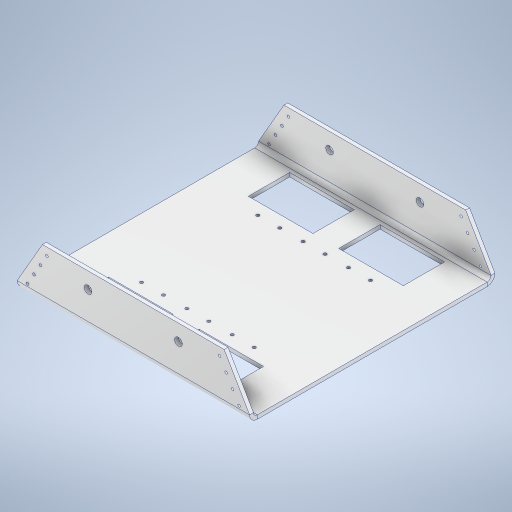
# Autodesk Inventor part: floor
Saved by Autodesk Inventor 2023 (Build 270158000, 158)
## iProperties
Created: 2022-05-09
Part Number: floor
Material: Aluminum 6061
Document SubType Name: Sheet Metal
Designer: Dan
Density: 2.7 g/cm^3
Sheet Metal Rule: Default_mm
Appearance: Aluminum - Flat
Mass: 314.843 g
Surface Area: 829.813 cm^2
Volume: 116.609 cm^3
Flat Pattern Width: 18 cm
Flat Pattern Length: 25.9572 cm
Flat Pattern Area: 467.229 cm^2
Sheet Metal Width: 180.000 mm
Sheet Metal Length: 259.572 mm
Sheet Metal Area: 46722.902 mm^2
Author: Dan
Autodesk Inventor part; units mm, degrees
ref_plane "YZ Plane" through (0, 0, 0) normal (1, 0, 0) x (0, 1, 0)
ref_plane "XZ Plane" through (0, 0, 0) normal (0, 1, 0) x (-1, 0, 0)
ref_plane "XY Plane" through (0, 0, 0) normal (0, 0, 1) x (1, 0, 0)
sketch "Sketch1" plane through (0, 0, 0) normal (0, 1, 0) x (-1, 0, 0)
  line L0 (0, 0) -> (90, 0)
  line L1 (90, 0) -> (90, -92)
  line L2 (90, -92) -> (0, -92)
  line L3 (0, -92) -> (0, 0)
  dimension "d0" = 92
  dimension "d1" = 90
  measures "d0" distance of L0.end L1.end
  measures "d1" distance of L1.end L2.end
extrude "Plate1" add sketch "Sketch1" along normal blind 3
sketch "Sketch2" plane through (0, 3, 0) normal (0, 0, 1) x (1, 0, 0)
  line L0 (-90, 0) -> (0, 0)
  line L1 (0, 0) -> (0, 37)
  line L2 (0, 37) -> (-90, 37)
  line L3 (-90, 37) -> (-90, 0)
  constraints: 6 end point, 1 horizontal, 1 perpendicular, 1 vertical
edge flange "Flange1" height 40 angle 90 thickness 3 bend radius 3 thickness toward (0, 0, 1) relief straight relief width 3 relief depth 1.5 edges at (-45, 3, 0) wall of the first edge with corners at (-90, 3, 0) (0, 3, 0) (0, 40, 0) (-90, 40, 0)
bend "Bend1"
corner "Corner1"
sketch "Sketch5" plane through (0, 3, 0) normal (0, 1, 0) x (1, 0, 0)
  line L0 (-80, 37.8978) -> (-30, 37.8978)
  line L1 (-30, 37.8978) -> (-30, 5.8978)
  line L2 (-30, 5.8978) -> (-80, 5.8978)
  line L3 (-80, 5.8978) -> (-80, 37.8978)
  line L4 (8.7792, 47.5) -> (-90, 47.5) construction
  line L5 (-90, 3) -> (-90, 92) projected
  line L6 (0, 92) -> (0, 3) projected
  line L7 (-55, 5.8978) -> (-55, 37.8978) construction
  point P0 (0, 0)
  dimension "d45" = 32
  dimension "d46" = 50
  dimension "d81" = 35
  constraints: 12 end point, 3 midpoint, 2 horizontal, 2 parallel, 1 perpendicular
  measures "d45" distance of L2.end L0.start
  measures "d46" distance of L1.end L2.end
  measures "d81" distance between parallel lines of L7 L5
extrude "Cut2" cut sketch "Sketch5" against normal blind 3
sketch "Sketch7" plane through (0, 3, 0) normal (0, 1, 0) x (1, 0, 0)
  line L0 (-90, 3) -> (-90, 92) projected
  line L1 (-80, 5.8978) -> (-80, 37.8978) projected
  line L2 (-80, 21.8978) -> (-101.6917, 21.8978) construction
  line L3 (-63.3842, 47) -> (-46.3842, 47) construction
  line L4 (-30, 37.8978) -> (-80, 37.8978) projected
  line L5 (-90, 92) -> (0, 92) projected
  point P0 (0, 0)
  point P1 (-81.5, 47)
  dimension "d88" = 17
  dimension "d90" = 45
  constraints: 4 end point, 2 horizontal, 1 horizontal alignment, 1 midpoint
  measures "d88" distance of L3.start L3.end
  measures "d90" distance from line of L5 point (-81.5, 47)
hole "Hole2" at (-46.3842, 3, -47) at (-63.3842, 3, -47) at (-81.5, 3, -47) direction (0, -1, 0) diameter 2.459 end through all thread size "M3x0.5" class "6H" standard "ISO Metric profile"
sketch "Sketch4" plane through (-15, 0, 3) normal (0, 0, 1) x (1, 0, 0)
  circle A0 centre (6.906, 8.0192) radius 1
  line L0 (17.454, -10.2505) -> (-9.0222, 35.6077) construction
  circle A1 centre (1.906, 16.6795) radius 1
  circle A2 centre (-3.094, 25.3397) radius 1
  circle A3 centre (-8.094, 34) radius 1
  line L1 (15, 0) -> (-75, 0) projected
  line L2 (15, 6) -> (15, 3) projected
  line L3 (15, 40) -> (15, 6) projected
  line L4 (15, 6) -> (15, 40)
  line L5 (15, 40) -> (-4.6299, 40)
  line L6 (-75, 40) -> (15, 40) projected
  line L7 (15, 0) -> (15, 6) projected
  line L8 (15, 6) -> (-4.6299, 40)
  circle A4 centre (-40, 27.5) radius 3
  line L9 (-65, 3) -> (-15, 3) construction
  line L10 (-40, 3) -> (-40, 27.5) construction
  point P0 (0, 34.7059)
  point P1 (15, 3)
  point P2 (-65, 3)
  dimension "d26" = 2
  dimension "d36" = 10
  dimension "d63" = 6
  dimension "d64" = 6
  dimension "d65" = 30
  dimension "d82" = 6
  dimension "d83" = 27.5
  constraints: 12 end point, 5 centre point, 3 coincident, 2 point on line, 2 vertical, 1 horizontal, 1 midpoint, 1 parallel, 8 other
  measures "d26" diameter of A0
  measures "d36" distance of A0.centre A1.centre
  measures "d63" distance between parallel lines of L8 L0
  measures "d64" distance from line of L6 A3.centre
  measures "d65" angle to the sketch y axis of L8
  measures "d82" diameter of A4
  measures "d83" distance from line of L1 A4.centre
extrude "Cut1" cut sketch "Sketch4" against normal up to next
mirror "Mirror1" about plane through (-90, 0, 0) normal (-1, 0, 0)
mirror "Mirror2" about plane through (-90, 0, -92) normal (0, 0, -1)
equation "\"d47\" = Thickness"
equation "\"d24\" = Thickness"
equation "\"d2\" = Thickness"
equation "\"d3\" = BendReliefWidth"
equation "\"d4\" = BendReliefDepth"
equation "\"d5\" = MinimumRemnant"
equation "\"d6\" = TransitionRadius"
equation "\"d9\" = BendRadius"
equation "\"d10\" = CornerReliefSize"
equation "\"d11\" = GapSize"
equation "\"d12\" = JacobiRadiusSize"
equation "\"BendRadius\" = Thickness"
equation "\"BendReliefWidth\" = Thickness"
equation "\"BendReliefDepth\" = 0.5 * Thickness"
equation "\"CornerReliefSize\" = 4 * Thickness"
equation "\"MinimumRemnant\" = 2 * Thickness"
equation "\"TransitionRadius\" = BendRadius"
equation "\"JacobiRadiusSize\" = BendRadius"
equation "\"GapSize\" = Thickness"
equation "\"Thickness\" = 3"
body "Solid1"
